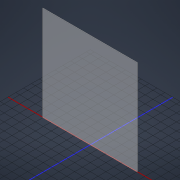
# Autodesk Inventor part: Panel Top
Saved by Autodesk Inventor 2022.2 (Build 262287010, 287A)
## iProperties
Created: 2022-03-16
Part Number: Panel Top
Material: Polycarbonat, klar
Document SubType Name: Modeling
Designer: sleib
Density: 1.2 g/cm^3
Appearance: Polycarbonat - klar
Author: sleib
Autodesk Inventor part; units mm, degrees
ref_plane "YZ Plane" through (0, 0, 0) normal (1, 0, 0) x (0, 1, 0)
ref_plane "XZ Plane" through (0, 0, 0) normal (0, 1, 0) x (-1, 0, 0)
ref_plane "XY Plane" through (0, 0, 0) normal (0, 0, 1) x (1, 0, 0)
sketch "Skizze1" plane through (0, 0, 0) normal (0, 0, 1) x (1, 0, 0)
  line L0 (-242, -242) -> (242, -242)
  line L1 (242, -242) -> (242, 242)
  line L2 (242, 242) -> (-242, 242)
  line L3 (-242, 242) -> (-242, -242)
  line L4 (-242, -242) -> (242, 242) construction
  line L5 (242, -242) -> (-242, 242) construction
  point P0 (0, 0)
  dimension "d0" = 484
  dimension "d1" = 484
  constraints: 12 end point, 2 midpoint, 2 parallel, 1 horizontal, 1 perpendicular
  measures "d0" distance of L1.end L2.end
  measures "d1" distance of L2.end L0.start
extrude "Extrusion1" add sketch "Skizze1" along normal blind 3
